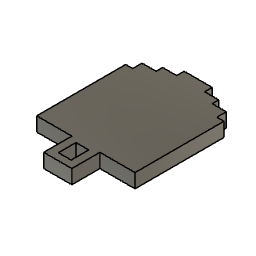
Keychain (Autodesk Fusion 360 design; units mm, degrees)
Autodesk Fusion 360 part; units mm, degrees
sketch "breloc" plane through (0, 0, 0) normal (0, 0, 1) x (1, 0, 0)
  line L0 (60, 60) -> (40, 60)
  line L1 (85, 80) -> (85, 140)
  line L2 (50, 160) -> (60, 160)
  line L3 (60, 160) -> (60, 154.6462)
  line L4 (60, 154.6462) -> (70, 154.6462)
  line L5 (70, 154.6462) -> (70, 150)
  line L6 (70, 150) -> (80, 150)
  line L7 (80, 150) -> (80, 143.3188)
  line L8 (80, 143.3188) -> (85, 143.3188)
  line L9 (85, 143.3188) -> (85, 140)
  line L10 (85, 80) -> (64.6572, 80)
  line L11 (15, 80) -> (15, 140)
  line L12 (40, 154.6462) -> (30, 154.6462)
  line L13 (50, 160) -> (40, 160)
  line L14 (30, 150) -> (20, 150)
  line L15 (20, 150) -> (20, 143.3188)
  line L16 (20, 143.3188) -> (15, 143.3188)
  line L17 (15, 143.3188) -> (15, 140)
  line L18 (30, 154.6462) -> (30, 150)
  line L19 (40, 160) -> (40, 154.6462)
  line L20 (15, 80) -> (35.3428, 80)
  line L21 (40, 80) -> (40, 60)
  line L22 (60, 80) -> (60, 60)
  line L23 (64.6572, 80) -> (60, 80)
  line L24 (40, 80) -> (35.3428, 80)
  line L25 (50, 80) -> (50, 77.5)
  line L26 (54.5281, 77.5) -> (54.5281, 65)
  line L27 (54.5281, 65) -> (50, 65)
  line L28 (54.5281, 77.5) -> (50, 77.5)
  line L29 (45.4719, 77.5) -> (45.4719, 65)
  line L30 (45.4719, 77.5) -> (50, 77.5)
  line L31 (45.4719, 65) -> (50, 65)
  dimension "d7" = 60
  constraint horizontal L0
  constraint vertical L1
  constraint perpendicular L2 L3
  constraint perpendicular L3 L4
  constraint perpendicular L4 L5
  constraint perpendicular L5 L6
  constraint perpendicular L4 L7
  constraint perpendicular L1 L8
  constraint perpendicular L8 L9
  constraint perpendicular L1 L10
  constraint perpendicular L0 L21
  constraint perpendicular L0 L22
  constraint perpendicular L22 L23
  constraint perpendicular L21 L24
  constraint perpendicular L0 L25
  constraint parallel L25 L26
  constraint perpendicular L25 L28
  measures "d7" distance of L1.end L1.start
extrude "Extrude4" add sketch "breloc" along normal blind 10
extrude "Extrude3" [suppressed]
moveface "MoveFace1" [suppressed]
extrude "Extrude1" [suppressed]
extrude "Extrude2" [suppressed]
named bodies: "breloc", "corp_breloc"
